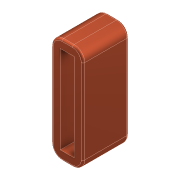
# Autodesk Inventor part: copper-wire
Saved by Autodesk Inventor 2022 (Build 260153000, 153)
## iProperties
Created: 2025-01-12
Part Number: copper-wire
Material: Generic
Document SubType Name: Modeling
Designer: Home
Density: 1 g/cm^3
Appearance: Copper - Satin
Author: Home
Autodesk Inventor part; units mm, degrees
ref_plane "YZ Plane" through (0, 0, 0) normal (1, 0, 0) x (0, 1, 0)
ref_plane "XZ Plane" through (0, 0, 0) normal (0, 1, 0) x (-1, 0, 0)
ref_plane "XY Plane" through (0, 0, 0) normal (0, 0, 1) x (1, 0, 0)
sketch "Sketch1" plane through (0, 0, 0) normal (0, 0, 1) x (1, 0, 0)
  line L0 (-2, -12.5) -> (2, -12.5)
  line L1 (2, -12.5) -> (2, 12.5)
  line L2 (2, 12.5) -> (-2, 12.5)
  line L3 (-2, 12.5) -> (-2, -12.5)
  line L4 (-2, -12.5) -> (2, 12.5) construction
  line L5 (2, -12.5) -> (-2, 12.5) construction
  line L6 (-4.5, -15) -> (4.5, -15)
  line L7 (4.5, -15) -> (4.5, 15)
  line L8 (4.5, 15) -> (-4.5, 15)
  line L9 (-4.5, 15) -> (-4.5, -15)
  line L10 (-4.5, -15) -> (4.5, 15) construction
  line L11 (4.5, -15) -> (-4.5, 15) construction
  point P0 (0, 0)
  dimension "d0" = 4
  dimension "d1" = 25
  dimension "d2" = 9
  dimension "d3" = 30
  constraints: 24 end point, 4 midpoint, 4 parallel, 2 horizontal, 2 perpendicular
  measures "d0" distance of L2.end L1.end
  measures "d1" distance of L1.end L0.end
  measures "d2" distance of L8.end L7.end
  measures "d3" distance of L7.end L6.end
extrude "Extrusion1" add sketch "Sketch1" along normal blind 13
fillet "Fillet1" radius 3 4 edges at (-4.5, 15, 6.5) (4.5, 15, 6.5) (4.5, -15, 6.5) (-4.5, -15, 6.5)
fillet "Fillet2" radius 0.5 16 edges at (-3.6213, 14.1213, 13) (-4.5, 0, 13) (-3.6213, -14.1213, 13) (0, -15, 13) (3.6213, -14.1213, 13) (4.5, 0, 13) (3.6213, 14.1213, 13) (0, 15, 13) (-3.6213, 14.1213, 0) (-4.5, 0, 0) (-3.6213, -14.1213, 0) (0, -15, 0) (3.6213, -14.1213, 0) (4.5, 0, 0) (3.6213, 14.1213, 0) (0, 15, 0)
body "Solid1"
